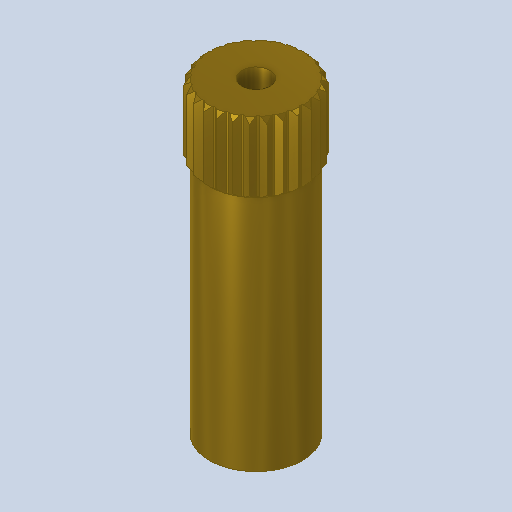
# Autodesk Inventor part: Eje
Saved by Autodesk Inventor 2023 (Build 270158000, 158)
## iProperties
Created: 2016-09-27
Part Number: Eje
Material: Aluminio 6061
Document SubType Name: Modeling
Designer: Julian
Density: 2.7 g/cm^3
Appearance: Metal 2400F(1)
Mass: 1.03301 g
Surface Area: 3.8433 cm^2
Volume: 0.382595 cm^3
Author: Julian
Autodesk Inventor part; units mm, degrees
ref_plane "YZ Plane" through (0, 0, 0) normal (1, 0, 0) x (0, 1, 0)
sketch "Boceto1" plane through (0, 0, 0) normal (0, 1, 0) x (-1, 0, 0)
  circle A0 centre (0, 0) radius 2.9
  dimension "d0" = 5.8
  constraints: 1 centre point, 1 coincident
  measures "d0" diameter of A0
extrude "Extrusión1" add sketch "Boceto1" along normal blind 13.5
sketch "Boceto2" plane through (0, 13.5, 0) normal (0, 1, 0) x (1, 0, 0)
  circle A0 centre (0, 0) radius 2.9 projected
  circle A1 centre (0, 0) radius 2.6
  dimension "d3" = 0.3
  constraints: 1 centre point
  measures "d3" radial gap between concentric circles of A0 A1
extrude "Extrusión2" add sketch "Boceto2" along normal blind 4 contours A1
sketch "Boceto3" plane through (0, 17.5, 0) normal (0, 1, 0) x (1, 0, 0)
  line L0 (-1.2753, 2.6045) -> (-1.1434, 2.3351)
  circle A0 centre (0, 0) radius 2.6 projected
  circle A1 centre (0, 0) radius 2.6 projected
  circle A2 centre (0, 0) radius 2.6 projected
  line L1 (-1.3737, 2.2075) -> (-1.2753, 2.6045)
  line L2 (-0.9014, 2.4387) -> (-1.2753, 2.6045)
  arc A3 (-0.9014, 2.4387) -> (-1.3737, 2.2075) centre (0, 0) ccw
  dimension "d21" = 0.3
  dimension "d22" = 80
  constraints: 7 point on circle, 6 end point, 1 centre point, 1 equal length, 3 other
  measures "d21" distance of L0.start L0.end
  measures "d22" angle of L2 L1
extrude "Extrusión3" add sketch "Boceto3" against normal blind 4 contours L2 A0 L0 | L0 A0 L1
pattern_circular "Patrón circular1" count 26 over 360 about axis through (0, 13.5, 0) along (0, 1, 0) of "Extrusión3"
ref_plane "Plano de trabajo1" through (1.8616, 17.5, 2.2236) normal (-0.766, 0, 0.6428) x (0, -1, 0)
sketch "Boceto5" plane through (1.8616, 17.5, 2.2236) normal (-0.766, 0, 0.6428) x (0, -1, 0)
  line L0 (0, -0.3136) -> (0, 0) projected
  line L1 (0, 0) -> (4, 0) projected
  line L2 (0, -0.25) -> (0.25, 0)
  line L3 (0, -0.25) -> (0.3536, -0.25) construction
  line L4 (0.25, 0) -> (0, 0)
  point P0 (17.5, -2.9)
  dimension "d25" = 45
  dimension "d26" = 0.25
  constraints: 6 end point, 2 point on line, 1 collinear, 1 equal length, 1 horizontal
  measures "d25" angle of L3 L2
  measures "d26" horizontal distance of L2.start L2.end
extrude "Extrusión4" cut sketch "Boceto5" along normal mid plane 0.7
pattern_circular "Patrón circular2" count 26 over 360 about axis through (0, 0, 0) along (0, 1, 0) of "Extrusión4"
sketch "Boceto6" plane through (0, 17.5, 0) normal (0, 1, 0) x (1, 0, 0)
  circle A0 centre (0, 0) radius 0.8
  dimension "d32" = 1.6
  constraints: 1 centre point, 1 coincident
  measures "d32" diameter of A0
extrude "Extrusión5" cut sketch "Boceto6" against normal blind 4
sketch "Boceto7" plane through (0, 0, 0) normal (0, -1, 0) x (1, 0, 0)
  circle A0 centre (0, 0) radius 2.9 projected
  circle A1 centre (0, 0) radius 2.65
  dimension "d38" = 5.3
  constraints: 1 centre point
  measures "d38" diameter of A1
extrude "Extrusión6" cut sketch "Boceto7" against normal blind 13.5
ref_plane "Plano de trabajo3" through (2.5999, 15.5, 0.022) normal (0, 1, 0) x (-1, 0, 0)
mirror "Simetría2" about plane through (2.5999, 15.5, 0.022) normal (0, 1, 0) of "Extrusión4", "Patrón circular2"
